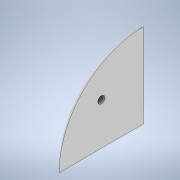
# Autodesk Inventor part: 3DPrintShapeCorner
Saved by Autodesk Inventor 2022 (Build 260153000, 153)
## iProperties
Created: 2022-04-20
Part Number: 3DPrintShapeCorner
Material: Generic
Document SubType Name: Modeling
Designer: Bruger
Density: 1 g/cm^3
Appearance: Default
Author: Bruger
Autodesk Inventor part; units mm, degrees
ref_plane "YZ Plane" through (0, 0, 0) normal (1, 0, 0) x (0, 1, 0)
ref_plane "XZ Plane" through (0, 0, 0) normal (0, 1, 0) x (-1, 0, 0)
ref_plane "XY Plane" through (0, 0, 0) normal (0, 0, 1) x (1, 0, 0)
sketch "Sketch1" plane through (0, 0, 0) normal (0, 1, 0) x (-1, 0, 0)
  line L0 (0, 0) -> (0, -150)
  line L1 (0, -150) -> (50, -150)
  line L2 (0, 0) -> (50, -44.9152) construction
  line L3 (50, -44.9152) -> (50, -150) construction
  spline S0 degree 2 poles (0, 0) (50, -44.9152) (50, -150) knots 1 1 1 2 2 2
  dimension "d0" = 150
  dimension "d2" = 50
  constraints: 4 end point, 1 horizontal, 1 vertical, 3 other
  measures "d0" distance of L0.start L0.end
  measures "d2" distance of L0.end L1.end
revolve "Revolution1" add sketch "Sketch1" angle 90 about axis through (0, 0, -150) along (-1, 0, 0)
sketch "Sketch2" plane through (0, 0, -150) normal (0, 0, -1) x (-1, 0, 0)
  line L0 (0, 150) -> (0, 0) projected
  line L1 (0, 0) -> (50, 0) projected
  line L2 (0, 0) -> (20, 0)
  line L3 (20, 0) -> (20, 50)
  line L4 (15, 55) -> (25, 55)
  line L5 (25, 55) -> (25, 45)
  line L6 (25, 45) -> (15, 45)
  line L7 (15, 45) -> (15, 55)
  line L8 (15, 55) -> (25, 45) construction
  line L9 (25, 55) -> (15, 45) construction
  dimension "d9" = 20
  dimension "d10" = 50
  dimension "d11" = 10
  dimension "d12" = 10
  constraints: 16 end point, 2 midpoint, 2 parallel, 2 perpendicular, 1 horizontal, 1 point on line
  measures "d9" distance of L0.end L2.end
  measures "d10" distance of L2.end L3.end
  measures "d11" distance of L5.end L6.end
  measures "d12" distance of L4.end L5.end
extrude "Extrusion1" add sketch "Sketch2" along normal blind 10
sketch "Sketch3" plane through (-50, 0, -150) normal (0, -1, 0) x (1, 0, 0)
  line L0 (50, 0) -> (30, 0)
  line L1 (50, 0) -> (0, 0) projected
  line L2 (30, 0) -> (30, 50)
  line L3 (35.1, 44.9) -> (24.9, 44.9)
  line L4 (24.9, 44.9) -> (24.9, 55.1)
  line L5 (24.9, 55.1) -> (35.1, 55.1)
  line L6 (35.1, 55.1) -> (35.1, 44.9)
  line L7 (35.1, 44.9) -> (24.9, 55.1) construction
  line L8 (24.9, 44.9) -> (35.1, 55.1) construction
  point P0 (50, 150)
  dimension "d19" = 20
  dimension "d20" = 50
  dimension "d21" = 10.2
  dimension "d22" = 10.2
  constraints: 16 end point, 2 midpoint, 2 parallel, 2 perpendicular, 1 horizontal, 1 point on line
  measures "d19" distance of L0.start L0.end
  measures "d20" distance of L0.end L2.end
  measures "d21" distance of L4.end L5.end
  measures "d22" distance of L3.end L4.end
extrude "Extrusion2" cut sketch "Sketch3" against normal blind 10
sketch "Sketch4" plane through (0, 0, 0) normal (1, 0, 0) x (0, 0, -1)
  line L0 (0, 0) -> (150, 0) projected
  line L1 (150, 0) -> (150, 75)
  line L2 (150, 150) -> (150, 0) projected
  line L3 (150, 75) -> (75, 75)
  circle A0 centre (75, 75) radius 6.25
  line L4 (75, 75) -> (75, 64)
  line L5 (75, 75) -> (84.5263, 69.5)
  line L6 (75, 75) -> (84.5263, 80.5)
  line L7 (75, 75) -> (75, 86)
  line L8 (75, 75) -> (65.4737, 80.5)
  line L9 (75, 75) -> (65.4737, 69.5)
  line L10 (75, 64) -> (65.4737, 69.5)
  line L11 (65.4737, 69.5) -> (65.4737, 80.5)
  line L12 (65.4737, 80.5) -> (75, 86)
  line L13 (75, 86) -> (84.5263, 80.5)
  line L14 (84.5263, 80.5) -> (84.5263, 69.5)
  line L15 (84.5263, 69.5) -> (75, 64)
  dimension "d25" = 75
  dimension "d26" = 75
  dimension "d27" = 12.5
  dimension "d33" = 11
  dimension "d36" = 360
  constraints: 28 end point, 3 parallel, 2 vertical, 1 centre point, 1 coincident, 1 midpoint, 1 perpendicular, 19 other
  measures "d25" distance of L0.end L1.end
  measures "d26" distance of L1.end L3.end
  measures "d27" diameter of A0
  measures "d33" distance of L4.start L4.end
extrude "Extrusion5" cut sketch "Sketch4" against normal blind 59.85
extrude "Extrusion6" add sketch "Sketch4" against normal blind 5 contours A0 L6 L14 L3 | L3 L14 L5 A0 | A0 L7 L13 L6 | L5 L15 L4 A0 | L4 L10 L9 A0 | A0 L8 L12 L7 | A0 L9 L11 L8
body "Solid1"
